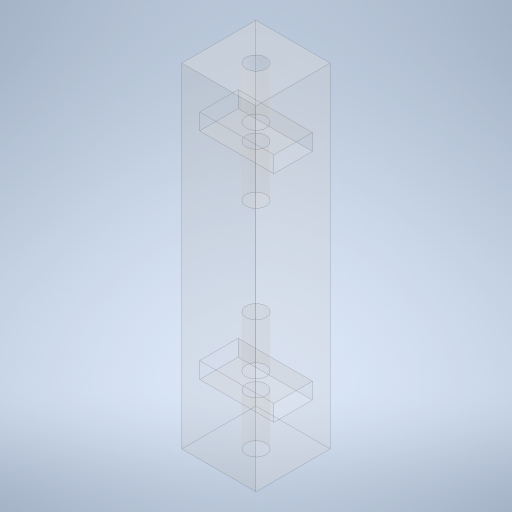
# Autodesk Inventor part: frame_head2
Saved by Autodesk Inventor 2024 (Build 280153000, 153)
## iProperties
Created: 2024-09-08
Part Number: frame_head2
Material: PMMA 플라스틱
Document SubType Name: Modeling
Designer: jmha0
Density: 1.188 g/cm^3
Appearance: 폴리카보네이트 - 선명
Author: jmha0
Autodesk Inventor part; units mm, degrees
ref_plane "YZ Plane" through (0, 0, 0) normal (1, 0, 0) x (0, 1, 0)
ref_plane "XZ Plane" through (0, 0, 0) normal (0, 1, 0) x (-1, 0, 0)
ref_plane "XY Plane" through (0, 0, 0) normal (0, 0, 1) x (1, 0, 0)
sketch "스케치1" plane through (0, 0, 0) normal (0, 1, 0) x (-1, 0, 0)
  line L0 (-5, 5) -> (5, 5)
  line L1 (5, 5) -> (5, -5)
  line L2 (5, -5) -> (-5, -5)
  line L3 (-5, -5) -> (-5, 5)
  line L4 (-5, 5) -> (5, -5) construction
  line L5 (5, 5) -> (-5, -5) construction
  circle A0 centre (0, 0) radius 1.35
  dimension "d0" = 10
  dimension "d1" = 10
  dimension "d2" = 2.7
  constraints: 12 end point, 2 midpoint, 2 parallel, 1 centre point, 1 coincident, 1 horizontal, 1 perpendicular
  measures "d0" distance of L1.end L2.end
  measures "d1" distance of L0.end L1.end
  measures "d2" diameter of A0
extrude "돌출1" add sketch "스케치1" along normal blind 45 contours L0 L1 L2 L3 | A0
sketch "스케치2" plane through (0, 0, 0) normal (0, -1, 0) x (1, 0, 0)
  circle A0 centre (0, 0) radius 1.35
  dimension "d5" = 2.7
  constraints: 1 centre point, 1 coincident
  measures "d5" diameter of A0
extrude "돌출2" cut sketch "스케치2" against normal blind 16
sketch "스케치3" plane through (0, 45, 0) normal (0, 1, 0) x (1, 0, 0)
  circle A0 centre (0, 0) radius 1.35
  dimension "d8" = 2.7
  constraints: 1 centre point, 1 coincident
  measures "d8" diameter of A0
extrude "돌출3" cut sketch "스케치3" against normal blind 16
sketch "스케치4" plane through (5, 0, 5) normal (1, 0, 0) x (0, 0, -1)
  line L0 (0, 45) -> (10, 45) projected
  line L1 (10, 45) -> (0, 45) projected
  line L2 (3.65, 45) -> (6.35, 45) projected
  line L3 (3.65, 29) -> (6.35, 29) projected
  line L4 (3.65, 45) -> (6.35, 45) projected
  line L5 (10, 45) -> (0, 45) projected
  line L6 (0, 45) -> (10, 45) projected
  line L7 (3.65, 29) -> (6.35, 29) projected
  line L8 (3.65, 29) -> (6.35, 29) projected
  line L9 (3.65, 45) -> (6.35, 45) projected
  line L10 (10, 0) -> (0, 0) projected
  line L11 (0, 0) -> (10, 0) projected
  line L12 (6.35, 0) -> (3.65, 0) projected
  line L13 (6.35, 16) -> (3.65, 16) projected
  line L14 (6.35, 0) -> (3.65, 0) projected
  line L15 (0, 0) -> (10, 0) projected
  line L16 (10, 0) -> (0, 0) projected
  line L17 (6.35, 16) -> (3.65, 16) projected
  line L18 (6.35, 16) -> (3.65, 16) projected
  line L19 (6.35, 0) -> (3.65, 0) projected
  line L20 (10, 0) -> (10, 45) projected
  line L21 (0, 0) -> (0, 45) projected
  line L22 (0, 0) -> (0, 45) projected
  line L23 (10, 0) -> (10, 45) projected
  line L24 (10, 0) -> (10, 45) projected
  line L25 (10, 0) -> (10, 45) projected
  line L26 (10, 0) -> (0, 0) projected
  line L27 (0, 0) -> (0, 45) projected
  line L28 (10, 45) -> (0, 45) projected
  line L29 (10, 0) -> (10, 45) projected
  line L30 (0, 0) -> (0, 45) projected
  line L31 (0, 0) -> (0, 45) projected
  line L32 (0, 0) -> (10, 0) projected
  line L33 (10, 0) -> (10, 45) projected
  line L34 (0, 45) -> (10, 45) projected
  line L35 (0, 0) -> (0, 45) projected
  line L36 (3.65, 45) -> (3.65, 29) projected
  line L37 (6.35, 45) -> (6.35, 29) projected
  line L38 (3.65, 0) -> (3.65, 16) projected
  line L39 (6.35, 0) -> (6.35, 16) projected
  line L40 (2.4, 38.1) -> (7.6, 38.1)
  line L41 (7.6, 38.1) -> (7.6, 35.9)
  line L42 (7.6, 35.9) -> (2.4, 35.9)
  line L43 (2.4, 35.9) -> (2.4, 38.1)
  line L44 (2.4, 38.1) -> (7.6, 35.9) construction
  line L45 (7.6, 38.1) -> (2.4, 35.9) construction
  line L46 (2.4, 6.9) -> (7.6, 6.9)
  line L47 (7.6, 6.9) -> (7.6, 9.1)
  line L48 (7.6, 9.1) -> (2.4, 9.1)
  line L49 (2.4, 9.1) -> (2.4, 6.9)
  line L50 (2.4, 6.9) -> (7.6, 9.1) construction
  line L51 (7.6, 6.9) -> (2.4, 9.1) construction
  point P0 (5, 0)
  point P1 (5, 37)
  point P2 (5, 8)
  dimension "d11" = 5.2
  dimension "d12" = 2.2
  dimension "d13" = 5.2
  dimension "d14" = 2.2
  constraints: 24 end point, 4 midpoint, 4 parallel, 2 horizontal, 2 perpendicular
  measures "d11" distance of L41.end L42.end
  measures "d12" distance of L40.end L41.end
  measures "d13" distance of L48.end L47.end
  measures "d14" distance of L47.end L46.end
extrude "돌출4" cut sketch "스케치4" against normal blind 16 contours L40 L37 L42 L36 | L36 L42 L43 L40 | L40 L41 L42 L37 | L46 L49 L48 L38 | L38 L48 L39 L46 | L39 L48 L47 L46
